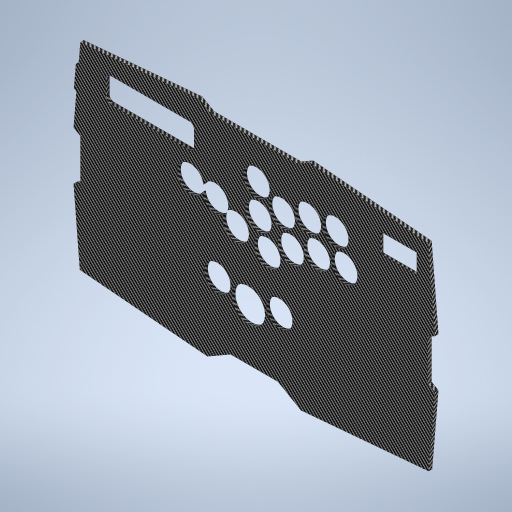
# Autodesk Inventor part: Top_Plate
Saved by Autodesk Inventor 2024 (Build 280153000, 153)
## iProperties
Created: 2023-09-20
Part Number: Top_Plate
Material: 常规
Document SubType Name: Modeling
Designer: nicx5
Density: 1 g/cm^3
Appearance: 碳纤维
Author: nicx5
Autodesk Inventor part; units mm, degrees
ref_plane "YZ Plane" through (0, 0, 0) normal (1, 0, 0) x (0, 1, 0)
ref_plane "XZ Plane" through (0, 0, 0) normal (0, 1, 0) x (-1, 0, 0)
ref_plane "XY Plane" through (0, 0, 0) normal (0, 0, 1) x (1, 0, 0)
derived "Frame.ipt"
sketch "top面板草图" plane through (0, 0, -3) normal (0, 0, 1) x (1, 0, 0)
  line L0 (-129.5, 55) -> (-52.5, 55)
  line L1 (-52.5, 55) -> (-52.5, 76.5)
  line L2 (-129.5, 76.5) -> (-52.5, 76.5)
  line L3 (-129.5, 55) -> (-129.5, 76.5)
  circle A0 centre (-55.7514, 33.4183) radius 11.5
  circle A1 centre (-34.0856, 29.598) radius 11.5
  circle A2 centre (-16.0643, 16.9793) radius 11.5
  circle A3 centre (-32.1234, -29.7121) radius 11.5
  circle A4 centre (-5.0643, -36.9094) radius 14.5
  circle A5 centre (21.9949, -29.7121) radius 11.5
  circle A6 centre (11.4783, 10.9768) radius 11.5
  circle A7 centre (3.7009, 34.6338) radius 11.5
  circle A8 centre (2.0127, 59.4994) radius 11.5
  circle A9 centre (24.0951, 47.2859) radius 11.5
  circle A10 centre (31.8725, 23.629) radius 11.5
  circle A11 centre (54.6939, 31.0574) radius 11.5
  circle A12 centre (46.9166, 54.7144) radius 11.5
  circle A13 centre (70.8507, 56.4914) radius 11.5
  circle A14 centre (78.628, 32.8344) radius 11.5
  line L4 (157.6336, 21.2378) -> (151.7356, 88.6532)
  line L5 (151.7356, 88.6532) -> (48.367, 97.6967)
  line L6 (48.367, 97.6967) -> (38.067, 91.75)
  line L7 (38.067, 91.75) -> (-38.067, 91.75)
  line L8 (-38.067, 91.75) -> (-48.367, 97.6967)
  line L9 (-48.367, 97.6967) -> (-151.7356, 88.6532)
  line L10 (-151.7356, 88.6532) -> (-153.2586, 71.2446)
  line L11 (-153.2586, 71.2446) -> (-154.5006, 70.2025)
  line L12 (157.6336, 21.2378) -> (151.75, 17.8409)
  line L13 (151.75, -17.8409) -> (157.6336, -21.2378)
  line L14 (157.6336, -21.2378) -> (152.1781, -83.5953)
  line L15 (-20.7465, -81.75) -> (20.7465, -81.75)
  line L16 (20.7465, -81.75) -> (40.8177, -93.3381)
  line L17 (40.8177, -93.3381) -> (152.1781, -83.5953)
  line L18 (-157.6336, -21.2378) -> (-152.1781, -83.5953)
  line L19 (-152.1781, -83.5953) -> (-40.8177, -93.3381)
  line L20 (-40.8177, -93.3381) -> (-20.7465, -81.75)
  line L21 (-157.6336, -21.2378) -> (-151.7501, -17.841)
  line L22 (-151.7501, 17.841) -> (-157.6336, 21.2378)
  line L23 (-157.6336, 21.2378) -> (-155.158, 49.5347)
  line L24 (-155.158, 49.5347) -> (-156.2001, 50.7767)
  line L25 (-154.5006, 70.2025) -> (-155.6, 70.2986)
  line L26 (-156.2001, 50.7767) -> (-157.2995, 50.8728)
  line L27 (-155.6, 70.2986) -> (-157.2995, 50.8728)
  line L28 (108.38, 83.05) -> (108.38, 48.65)
  line L29 (108.38, 48.65) -> (144.2, 48.65)
  line L30 (144.2, 48.65) -> (144.2, 83.05)
  line L31 (108.38, 83.05) -> (144.2, 83.05)
  line L32 (110.58, 59.8) -> (142, 59.8)
  line L33 (110.58, 59.8) -> (110.58, 76.5)
  line L34 (110.58, 76.5) -> (142, 76.5)
  line L35 (142, 59.8) -> (142, 76.5)
  line L36 (-151.7501, -17.841) -> (-151.7501, 17.841)
  line L37 (151.75, 17.8409) -> (151.75, -17.8409)
  point P0 (0, 0)
  point P1 (-154.577, 70.4647)
  point P2 (-156.3209, 50.5317)
  point P3 (-26.9988, 20.5412)
  point P4 (-45.5009, 28.205)
  point P5 (-44.3361, 34.8113)
  point P6 (-23.1511, 26.0362)
extrude "拉伸1" add sketch "top面板草图" along normal blind 3 contours L12 L37 L13 L14 L17 L16 L15 L20 L19 L18 L21 L36 L22 L23 L24 L26 L27 L25 L11 L10 L9 L8 L7 L6 L5 L4 | L31 L30 L29 L28
extrude "拉伸2" cut sketch "top面板草图" along normal blind 1 contours L31 L30 L29 L28
fillet "圆角1" radius 4 4 edges at (-129.5, 76.5, -1.5) (-129.5, 55, -1.5) (-52.5, 76.5, -1.5) (-52.5, 55, -1.5)
